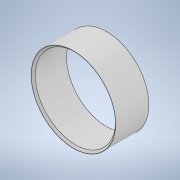
# Autodesk Inventor part: Part4
Saved by Autodesk Inventor 2020.2 (Build 242310000, 310)
## iProperties
Created: 2020-03-24
Part Number: Part4
Material: Generic
Document SubType Name: Modeling
Designer: iamin
Density: 1 g/cm^3
Appearance: Default
VLDS_Profile: Default Part
VLDS_TimeStamp: 2020-04-25
VLDS_FailCnt: 1
VLDS_AcceptCnt: 0
Author: iamin
## iProperties of the stored document _3DPrint.ipt
Created: 2020-04-25
Part Number: _3DPrint
Material: Generic
Document SubType Name: Modeling
Designer: iamin
Density: 1 g/cm^3
Appearance: Default
Author: iamin
Autodesk Inventor part; units mm, degrees
ref_plane "YZ Plane" through (0, 0, 0) normal (1, 0, 0) x (0, 1, 0)
ref_plane "XZ Plane" through (0, 0, 0) normal (0, 1, 0) x (-1, 0, 0)
ref_plane "XY Plane" through (0, 0, 0) normal (0, 0, 1) x (1, 0, 0)
sketch "Sketch1" plane through (0, 0, 0) normal (0, 0, 1) x (1, 0, 0)
  circle A0 centre (0, 0) radius 20.775
  circle A1 centre (0, 0) radius 19.6781
  dimension "d9" = 1.0969
  dimension "d10" = 41.55
  constraints: 2 centre point, 1 coincident
  measures "d9" radial gap between concentric circles of A0 A1
  measures "d10" diameter of A0
extrude "Extrusion1" add sketch "Sketch1" along normal mid plane 17.8
chamfer "Chamfer1" distance 1 angle 45 1 edges at (-19.6781, 0, 8.9)
sketch "Sketch2" plane through (0, 0, -8.9) normal (0, 0, -1) x (-1, 0, 0)
  circle A0 centre (0, 0) radius 21.8479
  constraints: 1 centre point, 1 coincident
extrude "Extrusion2" cut sketch "Sketch2" against normal blind 1.5
body "Solid1"
